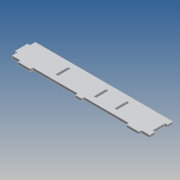
# Autodesk Inventor part: FixationBatterieLateral
Saved by Autodesk Inventor 2019 (Build 230136000, 136)
## iProperties
Created: 2019-08-27
Part Number: FixationBatterieLateral
Material: PVC-U
Document SubType Name: Modeling
Designer: jeremias.salamin
Density: 1.4 g/cm^3
Appearance: Lisse - Blanc
Description: FixationBatterieLateral
Author: jeremias.salamin
Autodesk Inventor part; units mm, degrees
ref_plane "YZ Plane" through (0, 0, 0) normal (1, 0, 0) x (0, 1, 0)
ref_plane "XZ Plane" through (0, 0, 0) normal (0, 1, 0) x (-1, 0, 0)
ref_plane "XY Plane" through (0, 0, 0) normal (0, 0, 1) x (1, 0, 0)
sketch "Sketch1" plane through (0, 0, 0) normal (0, 0, 1) x (1, 0, 0)
  line L0 (-62.09, 0) -> (62.09, 0) construction
  line L1 (0, 10.5) -> (0, -10.5) construction
  line L2 (44.35, -7.5) -> (-44.35, -7.5)
  line L3 (-44.35, -7.5) -> (-44.35, 7.5)
  line L4 (-44.35, 7.5) -> (44.35, 7.5)
  line L5 (44.35, 7.5) -> (44.35, -7.5)
  line L6 (44.35, -7.5) -> (-44.35, 7.5) construction
  line L7 (-44.35, -7.5) -> (44.35, 7.5) construction
  point P0 (0, 0)
  dimension "d0" = 88.7
  dimension "d1" = 15
  constraints: 12 end point, 2 midpoint, 2 parallel, 1 horizontal, 1 perpendicular
  measures "d0" distance of L3.end L4.end
  measures "d1" distance of L2.end L3.end
extrude "Extrusion1" add sketch "Sketch1" along normal mid plane 1.6
sketch "Esquisse2" plane through (0, 0, 0.8) normal (0, 0, 1) x (1, 0, 0)
  line L0 (-44.35, -7.5) -> (44.35, -7.5) construction
  line L1 (44.35, -7.5) -> (44.35, 7.5) construction
  line L2 (44.35, 7.5) -> (-44.35, 7.5) construction
  line L3 (-44.35, 7.5) -> (-44.35, -7.5) construction
  line L4 (0, 10.82) -> (0, -12.42) construction
  line L5 (-62.09, 0) -> (62.09, 0) construction
  line L6 (-39, -7.5) -> (-31, -7.5)
  line L7 (-31, -7.5) -> (-31, -9.1)
  line L8 (-31, -9.1) -> (-39, -9.1)
  line L9 (-39, -9.1) -> (-39, -7.5)
  line L10 (31, -7.5) -> (39, -7.5)
  line L11 (39, -7.5) -> (39, -9.1)
  line L12 (39, -9.1) -> (31, -9.1)
  line L13 (31, -9.1) -> (31, -7.5)
  line L14 (-2, -7.5) -> (2, -7.5)
  line L15 (2, -7.5) -> (2, -9.1)
  line L16 (2, -9.1) -> (-2, -9.1)
  line L17 (-2, -9.1) -> (-2, -7.5)
  point P0 (0, 0)
  dimension "d4" = 8
  dimension "d5" = 1.6
  dimension "d8" = 70
  dimension "d13" = 4
  dimension "d14" = 1.6
  constraints: 24 end point, 4 parallel, 3 horizontal, 2 perpendicular, 2 point on line, 10 other
  measures "d4" distance of L7.end L8.end
  measures "d5" distance of L6.end L7.end
  measures "d8" distance of L6.start L10.start
  measures "d13" distance of L15.end L16.end
  measures "d14" distance of L14.end L15.end
extrude "Extrusion2" add sketch "Esquisse2" against normal blind 1.6
sketch "Esquisse3" plane through (0, 0, 0.8) normal (0, 0, 1) x (1, 0, 0)
  line L0 (-44.35, -7.5) -> (-39, -7.5) construction
  line L1 (-39, -9.1) -> (-39, -7.5) construction
  line L2 (-31, -9.1) -> (-39, -9.1) construction
  line L3 (-31, -7.5) -> (-31, -9.1) construction
  line L4 (-31, -7.5) -> (-2, -7.5) construction
  line L5 (-2, -9.1) -> (-2, -7.5) construction
  line L6 (2, -9.1) -> (-2, -9.1) construction
  line L7 (2, -7.5) -> (2, -9.1) construction
  line L8 (2, -7.5) -> (31, -7.5) construction
  line L9 (31, -9.1) -> (31, -7.5) construction
  line L10 (39, -9.1) -> (31, -9.1) construction
  line L11 (39, -7.5) -> (39, -9.1) construction
  line L12 (39, -7.5) -> (44.35, -7.5) construction
  line L13 (44.35, -7.5) -> (44.35, 7.5) construction
  line L14 (44.35, 7.5) -> (-44.35, 7.5) construction
  line L15 (-44.35, 7.5) -> (-44.35, -7.5) construction
  line L16 (0, 10.82) -> (0, -12.42) construction
  line L17 (-64.01, 0) -> (62.41, 0) construction
  line L18 (-44.35, 4) -> (-45.95, 4)
  line L19 (-45.95, 4) -> (-45.95, -4)
  line L20 (-45.95, -4) -> (-44.35, -4)
  line L21 (-44.35, -4) -> (-44.35, 4)
  point P0 (0, 0)
  dimension "d17" = 1.6
  dimension "d18" = 8
  constraints: 8 end point, 2 parallel, 1 horizontal, 1 perpendicular, 1 point on line, 1 other
  measures "d17" distance of L20.end L19.end
  measures "d18" distance of L19.end L18.end
extrude "Extrusion3" add sketch "Esquisse3" against normal blind 1.6
sketch "Esquisse4" plane through (0, 0, 0.8) normal (0, 0, 1) x (1, 0, 0)
  line L0 (-18.25, -4) -> (-19.85, -4)
  line L1 (-19.85, -4) -> (-19.85, 4)
  line L2 (-19.85, 4) -> (-18.25, 4)
  line L3 (-18.25, 4) -> (-18.25, -4)
  line L4 (6.35, -4) -> (4.75, -4)
  line L5 (4.75, -4) -> (4.75, 4)
  line L6 (4.75, 4) -> (6.35, 4)
  line L7 (6.35, 4) -> (6.35, -4)
  line L8 (19.75, -4) -> (18.15, -4)
  line L9 (18.15, -4) -> (18.15, 4)
  line L10 (18.15, 4) -> (19.75, 4)
  line L11 (19.75, 4) -> (19.75, -4)
  line L12 (44.35, -4) -> (42.75, -4)
  line L13 (42.75, -4) -> (42.75, 4)
  line L14 (42.75, 4) -> (44.35, 4)
  line L15 (44.35, 4) -> (44.35, -4)
  point P0 (0, 0)
  constraints: 32 end point, 8 horizontal, 8 vertical, 16 other
extrude "Extrusion4" cut sketch "Esquisse4" against normal blind 1.6
